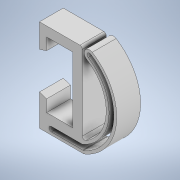
# Autodesk Inventor part: Clip
Saved by Autodesk Inventor 2022 (Build 260153000, 153)
## iProperties
Created: 2024-05-08
Part Number: Clip
Material: Generic
Document SubType Name: Modeling
Designer: Gotham City
Density: 1 g/cm^3
Appearance: Default
Author: Gotham City
Autodesk Inventor part; units mm, degrees
ref_plane "YZ Plane" through (0, 0, 0) normal (1, 0, 0) x (0, 1, 0)
ref_plane "XZ Plane" through (0, 0, 0) normal (0, 1, 0) x (-1, 0, 0)
ref_plane "XY Plane" through (0, 0, 0) normal (0, 0, 1) x (1, 0, 0)
sketch "Sketch1" plane through (0, 0, 0) normal (0, 0, 1) x (1, 0, 0)
  line L0 (14, 4) -> (14, 17.75)
  line L1 (14, 17.75) -> (18, 17.75) construction
  line L2 (18, 17.75) -> (18, 0)
  line L3 (3, 4) -> (3, 9)
  line L4 (3, 9) -> (0, 10)
  line L5 (3, 4) -> (14, 4)
  line L6 (14, 31.5) -> (14, 17.75)
  line L7 (18, 17.75) -> (18, 35.5)
  line L8 (3, 31.5) -> (3, 26.5)
  line L9 (3, 26.5) -> (0, 25.5)
  line L10 (3, 31.5) -> (14, 31.5)
  line L11 (-3.6, 0) -> (21.6, 0) construction
  line L12 (0, 35.5) -> (18, 35.5)
  line L13 (18, 0) -> (0, 0)
  line L14 (0, 35.5) -> (0, 25.5)
  line L15 (0, 0) -> (0, 10)
  dimension "d1" = 4
  dimension "d5" = 5
  dimension "d8" = 13.75
  dimension "d9" = 11
  dimension "d26" = 6
  dimension "d27" = 4
  dimension "d28" = 3
  constraints: 30 end point, 6 symmetric about line, 3 vertical, 1 collinear, 1 horizontal, 1 parallel, 1 point on line
  measures "d1" distance between parallel lines of L2 L0
  measures "d5" distance of L3.start L3.end
  measures "d8" distance between parallel lines of L1 L5
  measures "d9" distance between parallel lines of L0 L3
  measures "d26" vertical distance of L3.start L4.end
  measures "d27" distance between parallel lines of L5 L13
  measures "d28" distance between parallel lines of L15 L3
extrude "Extrusion1" add sketch "Sketch1" along normal blind 10
sketch "Sketch2" plane through (0, 0, 0) normal (0, 0, 1) x (1, 0, 0)
  circle A0 centre (23, 17.75) radius 5 construction
  line L0 (23, 17.75) -> (18, 17.75) construction
  arc A1 (18.6314, -3.2) -> (22.1621, 35.5) centre (10.6764, 17.0368) ccw
  arc A2 (18, 0) -> (20.4718, 32.7828) centre (10.6764, 17.0368) ccw
  arc A3 (18, 1.3146) -> (19.8379, 31.7639) centre (10.6764, 17.0368) ccw
  arc A4 (22.1621, 35.5) -> (19.8379, 31.7639) centre (21, 33.632) ccw
  arc A5 (21.5282, 34.4811) -> (20.4718, 32.7828) centre (21, 33.632) ccw
  line L1 (0, 0) -> (18, 0) projected
  line L2 (0, 2.0656) -> (0, 0)
  line L3 (18, 0) -> (18, 35.5) projected
  line L4 (18, 1.3146) -> (18, 0)
  line L5 (18, 0) -> (18, 35.5) projected
  arc A6 (18.4007, -2) -> (21.5282, 34.4811) centre (10.6764, 17.0368) ccw
  line L6 (0, 0) -> (18, 0) projected
  line L7 (18.4007, -2) -> (4, -2)
  line L8 (4, -2) -> (4, 0)
  line L9 (18.6314, -3.2) -> (0, -3.2)
  line L10 (0, -3.2) -> (0, 0)
  line L11 (29.1528, 15.4528) -> (31.1455, 15.282) construction
  dimension "d12" = 10
  dimension "d24" = 2.2
  dimension "d33" = 3
  dimension "d39" = 1.2
  dimension "d40" = 4
  dimension "d41" = 2
  dimension "d42" = 2
  dimension "d43" = 1.2
  constraints: 16 end point, 15 point on circle, 7 centre point, 6 tangent, 3 coincident, 3 horizontal, 2 perpendicular, 1 collinear, 1 horizontal alignment, 1 line through centre, 1 midpoint, 1 point on line, 1 vertical, 1 vertical alignment
  measures "d12" diameter of A0
  measures "d24" radius of A4
  measures "d33" distance from line of L3 A4.centre
  measures "d39" distance of A2.end A3.end
  measures "d40" distance between parallel lines of L8 L10
  measures "d41" distance between parallel lines of L1 L7
  measures "d42" distance of L11.start L11.end
  measures "d43" distance between parallel lines of L7 L9
extrude "Extrusion2" add sketch "Sketch2" along normal blind 10 contours L9 L10 L1 L8 L7 A6 A5 A2 L3 A3 A4 A1
fillet "Fillet3" radius 1 5 edges at (18, 1.3146, 5) (18.4007, -2, 5) (4, 0, 5) (4, -2, 5) (18.6314, -3.2, 5)
fillet "Fillet4" radius 1 1 edges at (18, 35.5, 5)
body "Solid1"
